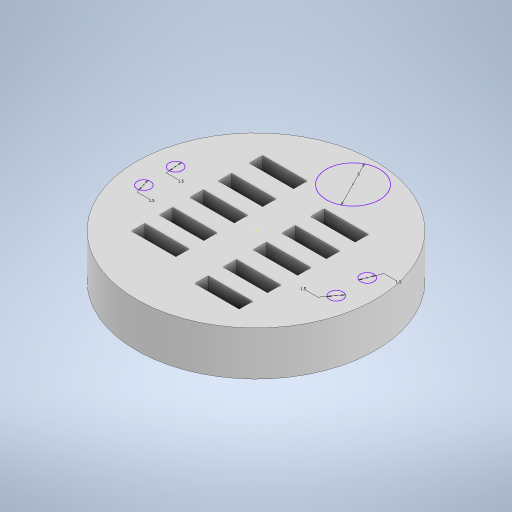
# Autodesk Inventor part: Seperator_BU
Saved by Autodesk Inventor 2023 (Build 270158000, 158)
## iProperties
Created: 2022-09-21
Part Number: Seperator_BU
Material: Generic
Document SubType Name: Modeling
Designer: Desmond
Density: 1 g/cm^3
Appearance: Default
Author: Desmond
Autodesk Inventor part; units mm, degrees
ref_plane "YZ Plane" through (0, 0, 0) normal (1, 0, 0) x (0, 1, 0)
ref_plane "XZ Plane" through (0, 0, 0) normal (0, 1, 0) x (-1, 0, 0)
ref_plane "XY Plane" through (0, 0, 0) normal (0, 0, 1) x (1, 0, 0)
sketch "Sketch3" plane through (0, 0, 0) normal (0, 1, 0) x (-1, 0, 0)
  circle A0 centre (0, 0) radius 13.5
  line L0 (-6.7499, 8.6501) -> (-1.7499, 8.6501)
  line L1 (-1.7499, 8.6501) -> (-1.7499, 7.1501)
  line L2 (-1.7499, 7.1501) -> (-6.7499, 7.1501)
  line L3 (-6.7499, 7.1501) -> (-6.7499, 8.6501)
  line L4 (-6.75, 5.45) -> (-1.7499, 5.45)
  line L5 (-1.7499, 5.45) -> (-1.7499, 3.95)
  line L6 (-1.7499, 3.95) -> (-6.75, 3.95)
  line L7 (-6.75, 3.95) -> (-6.75, 5.45)
  line L8 (-6.75, 2.0498) -> (-1.75, 2.0498)
  line L9 (-1.75, 2.0498) -> (-1.75, 0.5498)
  line L10 (-1.75, 0.5498) -> (-6.75, 0.5498)
  line L11 (-6.75, 0.5498) -> (-6.75, 2.0498)
  line L12 (-6.75, -1.2) -> (-1.75, -1.2)
  line L13 (-1.75, -1.2) -> (-1.75, -2.7)
  line L14 (-1.75, -2.7) -> (-6.75, -2.7)
  line L15 (-6.75, -2.7) -> (-6.75, -1.2)
  line L16 (-6.75, -4.4501) -> (-1.75, -4.4501)
  line L17 (-1.75, -4.4501) -> (-1.75, -5.9501)
  line L18 (-1.75, -5.9501) -> (-6.75, -5.9501)
  line L19 (-6.75, -5.9501) -> (-6.75, -4.4501)
  line L20 (1.9499, 7.1) -> (6.9499, 7.1)
  line L21 (6.9499, 7.1) -> (6.9499, 5.6)
  line L22 (6.9499, 5.6) -> (1.9499, 5.6)
  line L23 (1.9499, 5.6) -> (1.9499, 7.1)
  line L24 (1.9499, 3.95) -> (6.9499, 3.95)
  line L25 (6.9499, 3.95) -> (6.9499, 2.45)
  line L26 (6.9499, 2.45) -> (1.9499, 2.45)
  line L27 (1.9499, 2.45) -> (1.9499, 3.95)
  line L28 (1.9499, 0.5004) -> (6.9499, 0.5004)
  line L29 (6.9499, 0.5004) -> (6.9499, -0.9996)
  line L30 (6.9499, -0.9996) -> (1.9499, -0.9996)
  line L31 (1.9499, -0.9996) -> (1.9499, 0.5004)
  line L32 (1.9499, -2.7) -> (6.9499, -2.7)
  line L33 (6.9499, -2.7) -> (6.9499, -4.2)
  line L34 (6.9499, -4.2) -> (1.9499, -4.2)
  line L35 (1.9499, -4.2) -> (1.9499, -2.7)
  line L36 (1.9499, -6.1999) -> (6.9499, -6.1999)
  line L37 (6.9499, -6.1999) -> (6.9499, -7.6999)
  line L38 (6.9499, -7.6999) -> (1.9499, -7.6999)
  line L39 (1.9499, -7.6999) -> (1.9499, -6.1999)
  point P0 (-6.7499, 7.9001)
  point P1 (-6.75, 4.7)
  point P2 (-5.95, -5.2001)
  dimension "d3" = 27
  dimension "d4" = 5
  dimension "d5" = 1.5
  dimension "d6" = 1.5
  dimension "d7" = 5
  dimension "d8" = 1.5
  dimension "d9" = 5
  dimension "d10" = 1.5
  dimension "d11" = 5
  dimension "d12" = 1.5
  dimension "d13" = 0.8
  dimension "d14" = 5
  dimension "d15" = 1.5
  dimension "d16" = 5
  dimension "d17" = 1.5
  dimension "d18" = 5
  dimension "d19" = 1.5
  dimension "d20" = 5
  dimension "d21" = 1.5
  dimension "d22" = 1.5
  constraints: 80 end point, 20 parallel, 10 horizontal, 10 perpendicular, 3 point on line, 2 midpoint, 1 centre point
  measures "d3" diameter of A0
  measures "d4" distance of L1.end L2.end
  measures "d5" distance of L0.end L1.end
  measures "d6" distance of L4.end L5.end
  measures "d7" distance of L9.end L10.end
  measures "d8" distance of L8.end L9.end
  measures "d9" distance of L13.end L14.end
  measures "d10" distance of L12.end L13.end
  measures "d11" distance of L17.end L18.end
  measures "d12" distance of L16.end L17.end
  measures "d13" distance from line of L19 point (-5.95, -5.2)
  measures "d14" distance of L21.end L22.end
  measures "d15" distance of L20.end L21.end
  measures "d16" distance of L25.end L26.end
  measures "d17" distance of L24.end L25.end
  measures "d18" distance of L29.end L30.end
  measures "d19" distance of L28.end L29.end
  measures "d20" distance of L33.end L34.end
  measures "d21" distance of L32.end L33.end
  measures "d22" distance of L36.end L37.end
extrude "Extrusion1" add sketch "Sketch3" along normal blind 5
sketch "Sketch4" plane through (0, 5, 0) normal (0, 1, 0) x (1, 0, 0)
  circle A0 centre (-10.8, -1.9) radius 0.75
  circle A1 centre (-10.8, 1.7) radius 0.75
  circle A2 centre (10.9, -1.85) radius 0.75
  circle A3 centre (10.9, 1.65) radius 0.75
  circle A4 centre (0.958, 9.985) radius 3
  point P0 (0, 0)
  dimension "d25" = 1.5
  dimension "d26" = 1.5
  dimension "d27" = 1.5
  dimension "d28" = 1.5
  dimension "d29" = 6
  constraints: 5 centre point
  measures "d25" diameter of A0
  measures "d26" diameter of A1
  measures "d27" diameter of A2
  measures "d28" diameter of A3
  measures "d29" diameter of A4
body "Solid1"
